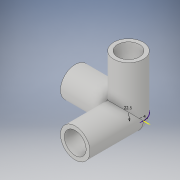
# Autodesk Inventor part: 3 axis end
Saved by Autodesk Inventor 2019 (Build 230136000, 136)
## iProperties
Created: 2018-10-04
Part Number: 3 axis end
Material: Generic
Document SubType Name: Modeling
Designer: HIVE
Density: 1 g/cm^3
Appearance: Default
Author: HIVE
Autodesk Inventor part; units mm, degrees
ref_plane "YZ Plane" through (0, 0, 0) normal (1, 0, 0) x (0, 1, 0)
ref_plane "XZ Plane" through (0, 0, 0) normal (0, 1, 0) x (-1, 0, 0)
ref_plane "XY Plane" through (0, 0, 0) normal (0, 0, 1) x (1, 0, 0)
sketch "Sketch1" plane through (0, 0, 0) normal (0, 1, 0) x (-1, 0, 0)
  circle A0 centre (0, 0) radius 11.25
  circle A1 centre (0, 0) radius 15.25
  line L0 (-15.25, 0) -> (15.25, 0)
  arc A2 (-15.25, 0) -> (15.25, 0) centre (0, 0) ccw
  line L1 (21.35, 0) -> (-21.35, 0) projected
  dimension "d0" = 22.5
  dimension "d1" = 4
  constraints: 4 point on circle, 3 centre point, 2 coincident, 2 end point, 1 horizontal
  measures "d0" diameter of A0
  measures "d1" radial gap between concentric circles of A0 A1
extrude "Extrusion1" add sketch "Sketch1" along normal blind 55 contours L0 A1 A0 | A0 L0 A1
extrude "Extrusion2" add sketch "Sketch1" along normal blind 15.25 contours L0 A0 | A0 L0
pattern_circular "Circular Pattern1" count 2 over 90 about axis through (-10, 0, 0) along (1, 0, 0) of "Extrusion1", "Extrusion2"
pattern_circular "Circular Pattern2" count 2 over 90 about axis through (0, 0, -10) along (0, 0, 1) of "Extrusion1", "Extrusion2"
revolve "Revolution1" add sketch "Sketch1" angle 360 about axis through (-10, 0, 0) along (1, 0, 0) picked at (13.66, -2.114) picked at (3.3205, -1.7427) contours L0 A1 A0 | A0 L0
equation "\"calc\" = 34.75"
body "Solid1"
